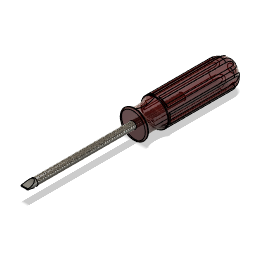
slot (Autodesk Fusion 360 design; units mm, degrees)
Autodesk Fusion 360 part; units mm, degrees
cylinder "CylinderPrimitive1" add diameter 28 height 100 placed x (1, 0, 0) y (0, 1, 0) z (0, 0, 1) at (0, 0, 0) makes body 1 in component "handle"
sketch "Sketch2" plane through (0, 0, 0) normal (0, 0, -1) x (-1, 0, 0) in component "handle"
  circle A0 centre (0, 0) radius 14
  circle A1 centre (-14, 0) radius 3
  dimension "d3" = 6
  constraint coincident A0 A1.centre
  measures "d3" diameter of A1
extrude "Extrude1" cut sketch "Sketch2" against normal blind 75 contours A0 A1 | A0 A1 picked at (-12.9761, 0) picked at (-14.9734, 0.0729) bodies 1 in component "handle"
pattern_circular "C-Pattern1" count 6 over 360 about axis through (0, 0, 1.75) along (0, 0, 1) of "Extrude1" in component "handle"
fillet "Fillet1" radius 10 6 edges at (0, 14, 0) (-12.1244, 7, 0) (-12.1244, -7, 0) (0, -14, 0) (12.1244, -7, 0) (12.1244, 7, 0) on bodies 1 in component "handle"
sketch "Sketch3" plane through (0, 0, 0) normal (1, 0, 0) x (0, 0, -1) in component "handle"
  ellipse E0 centre (-88, 15) end of major axis (-77.5, 15) minor radius 4
  line L0 (-98.5, 15) -> (-77.5, 15)
  line L1 (-88, 11) -> (-88, 19)
  dimension "d10" = 21
  dimension "d11" = 8
  constraint coincident E0 L0.start
  constraint coincident E0 L0.end
  constraint coincident E0 L1.start
  constraint coincident E0 L1.end
  constraint horizontal L0
  measures "d10" distance of E0
revolve "Revolve1" cut sketch "Sketch3" angle 360 about axis through (0, 0, 1.75) along (0, 0, 1) bodies 1 in component "handle"
fillet "Fillet2" radius 1.5 1 edges at (-13.0526, -5.0626, 100) on bodies 1 in component "handle"
fillet "Fillet3" radius 1 2 edges at (0.0058, -14, 77.8334) (0.006, -14, 98.1666) on bodies 1 in component "handle"
fillet "Fillet4" radius 2.5 18 edges at (-9.4224, 10.3546, 42.5) (-5.6106, 9.4655, 2.8619) (-4.2562, 13.3374, 42.5) (4.2562, 13.3374, 42.5) (5.3921, 9.5917, 2.8619) (9.4224, 10.3546, 42.5) (13.6786, 2.9827, 42.5) (11.0497, 0.5439, 2.921) (13.6786, -2.9827, 42.5) (9.4224, -10.3546, 42.5) (5.6106, -9.4655, 2.8619) (4.2562, -13.3374, 42.5) (-4.2562, -13.3374, 42.5) (-5.3921, -9.5917, 2.8619) (-9.4224, -10.3546, 42.5) (-13.6786, -2.9827, 42.5) (-11.0497, -0.5439, 2.921) (-13.6786, 2.9827, 42.5) on bodies 1 in component "handle"
fillet "Fillet5" radius 1 6 edges at (7, 12.1244, 75) (14, 0, 75) (7, -12.1244, 75) (-7, -12.1244, 75) (-14, 0, 75) (-7, 12.1244, 75) on bodies 1 in component "handle"
hole "Hole1" at (0, 0, 100) direction (0, 0, -1) diameter 7 depth 50 tip angle 180 bodies 1 in component "handle"
extrude "Extrude1'" add 1 faces at (0.9381, -0.555, 50) along direction (0, 0, 1) blind 150 separate body on bodies 1 makes body 2 in component "shank"
extrude "Extrude1''" add 1 faces at (0.9381, -0.555, 200) along direction (0, 0, 1) blind 10 separate body on bodies 2 makes body 3 in component "tip"
sketch "Sketch1" plane through (0, 0, 0) normal (1, 0, 0) x (0, 0, -1) in component "tip"
  arc A0 (-210, 0.5) -> (-201, 3.5) centre (-211.2799, 19.3396) ccw
  line L0 (-201, 3.5) -> (-210, 3.5)
  line L1 (-210, 3.5) -> (-210, 0.5)
  point P0 (-210, 0)
  dimension "d28" = 0.5
  dimension "d29" = 9
  constraint horizontal L0
  constraint perpendicular L0 L1
  measures "d28" distance of A0.start P0
  measures "d29" distance of A0.end L0.end
extrude "Extrude2" cut sketch "Sketch1" along normal through all and the other way through all bodies 3 in component "tip"
mirror "Mirror1" about plane through (0, 0, 0) normal (0, 1, 0) of "Extrude2" in component "tip"
component "handle" placed x (1, 0, 0) y (0, 1, 0) z (0, 0, 1) at (0, 0, 0)
component "shank" placed x (1, 0, 0) y (0, 1, 0) z (0, 0, 1) at (0, 0, 0)
component "tip" placed x (1, 0, 0) y (0, 1, 0) z (0, 0, 1) at (0, 0, 0)
named bodies: "cylinder", "slot head tip"
